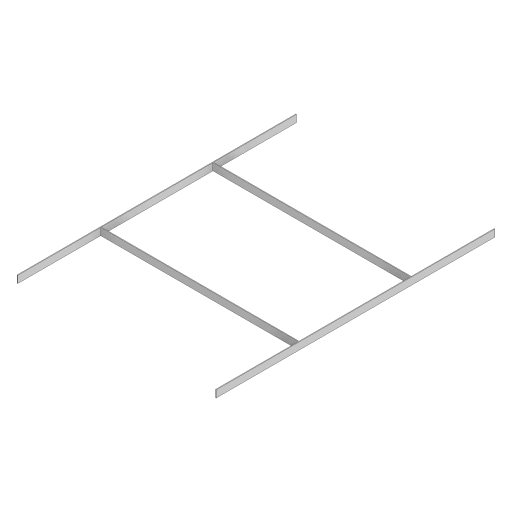
# Autodesk Inventor part: SOPORTE INERCIAL DE LA CAJA SEPARADORA
Saved by Autodesk Inventor 2024 (Build 280153000, 153)
## iProperties
Created: 2024-06-16
Part Number: SOPORTE INERCIAL DE LA CAJA SEPARADORA
Material: Generic
Document SubType Name: Modeling
Designer: Jhuliams
Density: 1 g/cm^3
Appearance: Default
Author: Jhuliams
Autodesk Inventor part; units mm, degrees
ref_plane "YZ Plane" through (0, 0, 0) normal (1, 0, 0) x (0, 1, 0)
ref_plane "XZ Plane" through (0, 0, 0) normal (0, 1, 0) x (-1, 0, 0)
ref_plane "XY Plane" through (0, 0, 0) normal (0, 0, 1) x (1, 0, 0)
sketch "Sketch1" plane through (0, 0, 0) normal (0, 1, 0) x (-1, 0, 0)
  line L0 (345, 196.12) -> (-345, 196.12)
  line L1 (-345, 196.12) -> (-345, -196.12)
  line L2 (-345, -196.12) -> (345, -196.12)
  line L3 (345, -196.12) -> (345, 196.12)
  line L4 (345, 196.12) -> (-345, -196.12) construction
  line L5 (-345, 196.12) -> (345, -196.12) construction
  line L6 (347.5, -198.62) -> (-347.5, -198.62)
  line L7 (-347.5, -198.62) -> (-347.5, 198.62)
  line L8 (-347.5, 198.62) -> (347.5, 198.62)
  line L9 (347.5, 198.62) -> (347.5, -198.62)
  line L10 (345, -196.12) -> (347.5, -196.12)
  line L11 (345, 196.12) -> (347.5, 196.12)
  line L12 (-345, -196.12) -> (-347.5, -196.12)
  line L13 (-345, 196.12) -> (-347.5, 196.12)
  point P0 (0, 0)
  dimension "d0" = 690
  dimension "d1" = 392.24
  dimension "d2" = 2.5
  constraints: 28 end point, 6 point on line, 4 parallel, 4 perpendicular, 2 midpoint, 1 horizontal, 3 other
  measures "d0" distance of L2.end L1.end
  measures "d1" distance of L1.end L0.end
  measures "d2" distance between parallel lines of L2 L6
extrude "Extrusion1" add sketch "Sketch1" along normal blind 25 contours L0 L13 L7 L8 L9 L11 | L10 L9 L6 L7 L12 L2
sketch "Sketch2" plane through (347.5, 0, 198.62) normal (1, 0, 0) x (0, 0, -1)
  line L0 (-291.38, 25) -> (688.62, 25)
  line L1 (688.62, 25) -> (688.62, -25)
  line L2 (688.62, -25) -> (-291.38, -25)
  line L3 (-291.38, -25) -> (-291.38, 25)
  line L4 (-291.38, 25) -> (688.62, -25) construction
  line L5 (688.62, 25) -> (-291.38, -25) construction
  line L6 (-291.38, 0) -> (688.62, 0)
  point P0 (198.62, 0)
  dimension "d5" = 980
  dimension "d6" = 50
  constraints: 14 end point, 4 midpoint, 2 parallel, 1 horizontal, 1 perpendicular
  measures "d5" distance of L1.end L2.end
  measures "d6" distance of L0.end L1.end
extrude "Extrusion2" add sketch "Sketch2" along normal blind 2.5 contours L0 L1 L6 L3
mirror "Mirror1" about plane through (0, 0, 0) normal (1, 0, 0) of "Extrusion2"
body "Solid1"
